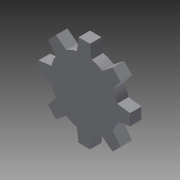
# Autodesk Inventor part: Planet
Saved by Autodesk Inventor 2013 (Build 170138000, 138)
## iProperties
Created: 2014-02-12
Part Number: Planet
Material: Generic
Document SubType Name: Modeling
Designer: robotics
Density: 1 g/cm^3
Author: robotics
Autodesk Inventor part; units mm, degrees
ref_plane "YZ Plane" through (0, 0, 0) normal (1, 0, 0) x (0, 1, 0)
ref_plane "XZ Plane" through (0, 0, 0) normal (0, 1, 0) x (-1, 0, 0)
ref_plane "XY Plane" through (0, 0, 0) normal (0, 0, 1) x (1, 0, 0)
sketch "Sketch1" plane through (0, 0, 0) normal (0, 0, 1) x (1, 0, 0)
  line L0 (0, 0) -> (0, 8.0538) construction
  line L1 (1.0291, 4.5587) -> (0.7937, 6.3467)
  line L2 (0.7937, 6.3467) -> (0, 6.3467)
  line L3 (-1.0291, 4.5587) -> (-0.7937, 6.3467)
  line L4 (-0.7937, 6.3467) -> (0, 6.3467)
  line L5 (-0.7937, 6.3467) -> (0.7937, 6.3467)
  line L6 (-2.4958, 3.9512) -> (-3.9265, 5.0491)
  line L7 (-3.9512, 2.4958) -> (-5.0491, 3.9265)
  line L8 (-5.0491, 3.9265) -> (-3.9265, 5.0491)
  line L9 (-4.5587, 1.0291) -> (-6.3467, 0.7938)
  line L10 (-4.5587, -1.0291) -> (-6.3467, -0.7937)
  line L11 (-6.3467, -0.7937) -> (-6.3467, 0.7938)
  line L12 (-3.9512, -2.4958) -> (-5.0491, -3.9265)
  line L13 (-2.4958, -3.9512) -> (-3.9265, -5.0491)
  line L14 (-3.9265, -5.0491) -> (-5.0491, -3.9265)
  line L15 (-1.0291, -4.5587) -> (-0.7938, -6.3467)
  line L16 (1.0291, -4.5587) -> (0.7937, -6.3467)
  line L17 (0.7937, -6.3467) -> (-0.7938, -6.3467)
  line L18 (2.4958, -3.9512) -> (3.9265, -5.0491)
  line L19 (3.9512, -2.4958) -> (5.0491, -3.9265)
  line L20 (5.0491, -3.9265) -> (3.9265, -5.0491)
  line L21 (4.5587, -1.0291) -> (6.3467, -0.7938)
  line L22 (4.5587, 1.0291) -> (6.3467, 0.7937)
  line L23 (6.3467, 0.7937) -> (6.3467, -0.7938)
  line L24 (3.9512, 2.4958) -> (5.0491, 3.9265)
  line L25 (2.4958, 3.9512) -> (3.9265, 5.0491)
  line L26 (3.9265, 5.0491) -> (5.0491, 3.9265)
  line L27 (-2.4958, 3.9512) -> (-1.0291, 4.5587) construction
  arc A0 (-3.9512, 2.4958) -> (-4.5587, 1.0291) centre (0, 0) ccw
  arc A1 (-1.0291, 4.5587) -> (-2.4958, 3.9512) centre (0, 0) ccw
  arc A2 (2.4958, 3.9512) -> (1.0291, 4.5587) centre (0, 0) ccw
  arc A3 (4.5587, 1.0291) -> (3.9512, 2.4958) centre (0, 0) ccw
  arc A4 (3.9512, -2.4958) -> (4.5587, -1.0291) centre (0, 0) ccw
  arc A5 (1.0291, -4.5587) -> (2.4958, -3.9512) centre (0, 0) ccw
  arc A6 (-4.5587, -1.0291) -> (-3.9512, -2.4958) centre (0, 0) ccw
  arc A7 (-2.4958, -3.9512) -> (-1.0291, -4.5587) centre (0, 0) ccw
  dimension "d0" = 1.5875
  dimension "d2" = 1.8034
  dimension "d7" = 120
  constraints: 56 end point, 16 point on circle, 8 centre point, 2 symmetric about line, 1 coincident, 1 collinear, 1 equal length, 1 perpendicular, 1 point on line, 1 vertical, 57 other
  measures "d0" distance of L4.start L1.end
  measures "d2" distance of L1.start L1.end
  measures "d7" angle of L3 L27
extrude "Extrusion1" add sketch "Sketch1" along normal blind 1.5875
body "Solid1"
